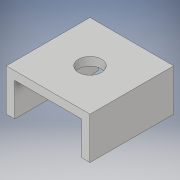
# Autodesk Inventor part: base
Saved by Autodesk Inventor 2019 (Build 230136000, 136)
## iProperties
Created: 2018-12-13
Part Number: base
Material: Generic
Document SubType Name: Modeling
Designer: garstka1245
Density: 1 g/cm^3
Appearance: Default
Author: garstka1245
Autodesk Inventor part; units mm, degrees
ref_plane "YZ Plane" through (0, 0, 0) normal (1, 0, 0) x (0, 1, 0)
ref_plane "XZ Plane" through (0, 0, 0) normal (0, 1, 0) x (-1, 0, 0)
ref_plane "XY Plane" through (0, 0, 0) normal (0, 0, 1) x (1, 0, 0)
sketch "Sketch1" plane through (0, 0, 0) normal (0, 1, 0) x (-1, 0, 0)
  line L0 (0, 0) -> (127, 0)
  line L1 (127, 0) -> (127, -127)
  line L2 (127, -127) -> (0, -127)
  line L3 (0, -127) -> (0, 0)
  circle A0 centre (63.5, -63.5) radius 17.4625
  dimension "d0" = 127
  dimension "d1" = 127
  dimension "d2" = 34.925
  constraints: 8 end point, 2 parallel, 1 centre point, 1 horizontal, 1 perpendicular
  measures "d0" distance of L1.end L2.end
  measures "d1" distance of L0.end L1.end
  measures "d2" diameter of A0
extrude "Extrusion1" add sketch "Sketch1" along normal blind 12.7
sketch "Sketch2" plane through (0, 0, 0) normal (0, -1, 0) x (1, 0, 0)
  line L0 (0, -127) -> (-127, -127) projected
  line L1 (-114.3, -127) -> (-114.3, 0)
  line L2 (-127, 0) -> (0, 0) projected
  line L3 (-12.7, 0) -> (-12.7, -127)
  line L4 (-127, 0) -> (-127, -127) projected
  line L5 (0, -127) -> (0, 0) projected
  dimension "d5" = 12.7
  dimension "d6" = 12.7
  constraints: 4 end point, 3 point on line, 1 perpendicular, 1 vertical
  measures "d5" distance between parallel lines of L4 L1
  measures "d6" distance between parallel lines of L5 L3
extrude "Extrusion2" add sketch "Sketch2" along normal blind 50.8 contours L0 L3 L2 L5 | L0 L4 L2 L1
equation "\"d1\" = d0"
body "Solid1"
